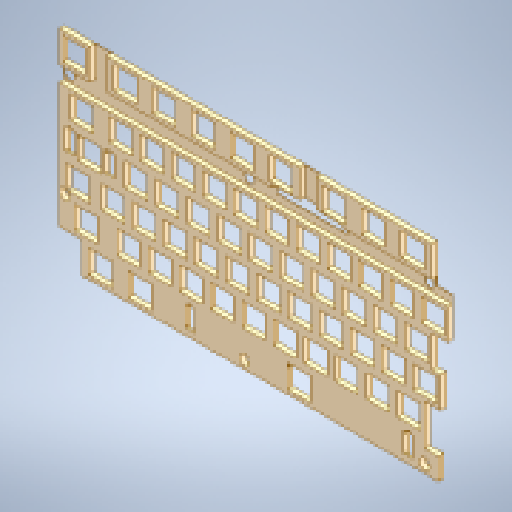
# Autodesk Inventor part: Left Plate
Saved by Autodesk Inventor 2025 (Build 290162000, 162)
## iProperties
Created: 2024-07-10
Part Number: Left Plate
Material: PET Plastic
Document SubType Name: Modeling
Designer: adam
Density: 1.541 g/cm^3
Appearance: Smooth - Off-White
Author: adam
Autodesk Inventor part; units mm, degrees
(part 1 of 3)
ref_plane "YZ Plane" through (0, 0, 0) normal (1, 0, 0) x (0, 1, 0)
ref_plane "XZ Plane" through (0, 0, 0) normal (0, 1, 0) x (-1, 0, 0)
ref_plane "XY Plane" through (0, 0, 0) normal (0, 0, 1) x (1, 0, 0)
sketch "Sketch5" plane through (0, 0, 0) normal (0, 0, 1) x (1, 0, 0)
  line L0 (-225, -62.5) -> (225, -62.5) construction
  line L1 (225, -62.5) -> (225, 62.5) construction
  line L2 (225, 62.5) -> (-225, 62.5) construction
  line L3 (-225, 62.5) -> (-225, -62.5) construction
  spline S0 degree 3 poles (89.83, -35.8909) (88.6584, -35.8909) (87.7087, -34.9412) (87.7087, -33.7696) knots 0 0 0 0 1 1 1 1 construction
  spline S1 degree 3 poles (87.7087, -33.7696) (87.7087, -32.598) (88.6584, -31.6483) (89.83, -31.6483) knots 0 0 0 0 1 1 1 1 construction
  arc A0 (91.9513, -33.7696) -> (89.83, -31.6483) centre (89.83, -33.7696) ccw construction
  spline S2 degree 3 poles (91.9513, -33.7696) (91.9513, -34.9412) (91.0016, -35.8909) (89.83, -35.8909) knots 0 0 0 0 1 1 1 1 construction
  arc A1 (215.8301, -43.274) -> (213.7088, -41.1527) centre (213.7088, -43.274) ccw construction
  spline S3 degree 3 poles (215.8301, -43.274) (215.8301, -44.4456) (214.8804, -45.3953) (213.7088, -45.3953) knots 0 0 0 0 1 1 1 1 construction
  spline S4 degree 3 poles (213.7088, -45.3953) (212.5372, -45.3953) (211.5875, -44.4456) (211.5875, -43.274) knots 0 0 0 0 1 1 1 1 construction
  spline S5 degree 3 poles (211.5875, -43.274) (211.5875, -42.1024) (212.5372, -41.1527) (213.7088, -41.1527) knots 0 0 0 0 1 1 1 1 construction
  arc A2 (196.7801, -33.722) -> (194.6588, -31.6007) centre (194.6588, -33.722) ccw construction
  spline S6 degree 3 poles (196.7801, -33.722) (196.7801, -34.58) (196.2633, -35.3535) (195.4706, -35.6818) knots 0 0 0 0 1 1 1 1 construction
  spline S7 degree 3 poles (195.4706, -35.6818) (194.6779, -36.0102) (193.7655, -35.8287) (193.1588, -35.222) knots 0 0 0 0 1 1 1 1 construction
  spline S8 degree 3 poles (193.1588, -35.222) (192.5521, -34.6153) (192.3706, -33.7029) (192.699, -32.9102) knots 0 0 0 0 1 1 1 1 construction
  spline S9 degree 3 poles (192.699, -32.9102) (193.0273, -32.1175) (193.8008, -31.6007) (194.6588, -31.6007) knots 0 0 0 0 1 1 1 1 construction
  arc A3 (196.7801, -52.772) -> (194.6588, -50.6507) centre (194.6588, -52.772) ccw construction
  spline S10 degree 3 poles (196.7801, -52.772) (196.7801, -53.63) (196.2633, -54.4035) (195.4706, -54.7318) knots 0 0 0 0 1 1 1 1 construction
  spline S11 degree 3 poles (195.4706, -54.7318) (194.6779, -55.0602) (193.7655, -54.8787) (193.1588, -54.272) knots 0 0 0 0 1 1 1 1 construction
  spline S12 degree 3 poles (193.1588, -54.272) (192.5521, -53.6653) (192.3706, -52.7529) (192.699, -51.9602) knots 0 0 0 0 1 1 1 1 construction
  spline S13 degree 3 poles (192.699, -51.9602) (193.0273, -51.1675) (193.8008, -50.6507) (194.6588, -50.6507) knots 0 0 0 0 1 1 1 1 construction
  arc A4 (215.8301, -14.672) -> (213.7088, -12.5507) centre (213.7088, -14.672) ccw construction
  spline S14 degree 3 poles (215.8301, -14.672) (215.8301, -15.53) (215.3133, -16.3035) (214.5206, -16.6318) knots 0 0 0 0 1 1 1 1 construction
  spline S15 degree 3 poles (214.5206, -16.6318) (213.7279, -16.9602) (212.8155, -16.7787) (212.2088, -16.172) knots 0 0 0 0 1 1 1 1 construction
  spline S16 degree 3 poles (212.2088, -16.172) (211.6021, -15.5653) (211.4206, -14.6529) (211.749, -13.8602) knots 0 0 0 0 1 1 1 1 construction
  spline S17 degree 3 poles (211.749, -13.8602) (212.0773, -13.0675) (212.8508, -12.5507) (213.7088, -12.5507) knots 0 0 0 0 1 1 1 1 construction
  arc A5 (196.7801, -14.672) -> (194.6588, -12.5507) centre (194.6588, -14.672) ccw construction
  spline S18 degree 3 poles (196.7801, -14.672) (196.7801, -15.53) (196.2633, -16.3035) (195.4706, -16.6318) knots 0 0 0 0 1 1 1 1 construction
  spline S19 degree 3 poles (195.4706, -16.6318) (194.6779, -16.9602) (193.7655, -16.7787) (193.1588, -16.172) knots 0 0 0 0 1 1 1 1 construction
  spline S20 degree 3 poles (193.1588, -16.172) (192.5521, -15.5653) (192.3706, -14.6529) (192.699, -13.8602) knots 0 0 0 0 1 1 1 1 construction
  spline S21 degree 3 poles (192.699, -13.8602) (193.0273, -13.0675) (193.8008, -12.5507) (194.6588, -12.5507) knots 0 0 0 0 1 1 1 1 construction
  spline S22 degree 3 poles (211.749, 5.1898) (212.0773, 5.9825) (212.8508, 6.4993) (213.7088, 6.4993) knots 0 0 0 0 1 1 1 1 construction
  arc A6 (215.8301, 4.378) -> (213.7088, 6.4993) centre (213.7088, 4.378) ccw construction
  spline S23 degree 3 poles (215.8301, 4.378) (215.8301, 3.52) (215.3133, 2.7465) (214.5206, 2.4182) knots 0 0 0 0 1 1 1 1 construction
  spline S24 degree 3 poles (214.5206, 2.4182) (213.7279, 2.0898) (212.8155, 2.2713) (212.2088, 2.878) knots 0 0 0 0 1 1 1 1 construction
  spline S25 degree 3 poles (212.2088, 2.878) (211.6021, 3.4847) (211.4206, 4.3971) (211.749, 5.1898) knots 0 0 0 0 1 1 1 1 construction
  arc A7 (196.7801, 4.378) -> (194.6588, 6.4993) centre (194.6588, 4.378) ccw construction
  spline S26 degree 3 poles (196.7801, 4.378) (196.7801, 3.52) (196.2633, 2.7465) (195.4706, 2.4182) knots 0 0 0 0 1 1 1 1 construction
  spline S27 degree 3 poles (195.4706, 2.4182) (194.6779, 2.0898) (193.7655, 2.2713) (193.1588, 2.878) knots 0 0 0 0 1 1 1 1 construction
  spline S28 degree 3 poles (193.1588, 2.878) (192.5521, 3.4847) (192.3706, 4.3971) (192.699, 5.1898) knots 0 0 0 0 1 1 1 1 construction
  spline S29 degree 3 poles (192.699, 5.1898) (193.0273, 5.9825) (193.8008, 6.4993) (194.6588, 6.4993) knots 0 0 0 0 1 1 1 1 construction
  spline S30 degree 3 poles (176.4206, 21.4682) (175.6279, 21.1398) (174.7155, 21.3213) (174.1088, 21.928) knots 0 0 0 0 1 1 1 1 construction
  spline S31 degree 3 poles (174.1088, 21.928) (173.5021, 22.5347) (173.3206, 23.4471) (173.649, 24.2398) knots 0 0 0 0 1 1 1 1 construction
  spline S32 degree 3 poles (173.649, 24.2398) (173.9773, 25.0325) (174.7508, 25.5493) (175.6088, 25.5493) knots 0 0 0 0 1 1 1 1 construction
  arc A8 (177.7301, 23.428) -> (175.6088, 25.5493) centre (175.6088, 23.428) ccw construction
  spline S33 degree 3 poles (177.7301, 23.428) (177.7301, 22.57) (177.2133, 21.7965) (176.4206, 21.4682) knots 0 0 0 0 1 1 1 1 construction
  spline S34 degree 3 poles (193.1588, 21.928) (192.5521, 22.5347) (192.3706, 23.4471) (192.699, 24.2398) knots 0 0 0 0 1 1 1 1 construction
  spline S35 degree 3 poles (192.699, 24.2398) (193.0273, 25.0325) (193.8008, 25.5493) (194.6588, 25.5493) knots 0 0 0 0 1 1 1 1 construction
  arc A9 (196.7801, 23.428) -> (194.6588, 25.5493) centre (194.6588, 23.428) ccw construction
  spline S36 degree 3 poles (196.7801, 23.428) (196.7801, 22.57) (196.2633, 21.7965) (195.4706, 21.4682) knots 0 0 0 0 1 1 1 1 construction
  spline S37 degree 3 poles (195.4706, 21.4682) (194.6779, 21.1398) (193.7655, 21.3213) (193.1588, 21.928) knots 0 0 0 0 1 1 1 1 construction
  arc A10 (215.8301, 23.428) -> (213.7088, 25.5493) centre (213.7088, 23.428) ccw construction
  spline S38 degree 3 poles (215.8301, 23.428) (215.8301, 22.57) (215.3133, 21.7965) (214.5206, 21.4682) knots 0 0 0 0 1 1 1 1 construction
  spline S39 degree 3 poles (214.5206, 21.4682) (213.7279, 21.1398) (212.8155, 21.3213) (212.2088, 21.928) knots 0 0 0 0 1 1 1 1 construction
  spline S40 degree 3 poles (212.2088, 21.928) (211.6021, 22.5347) (211.4206, 23.4471) (211.749, 24.2398) knots 0 0 0 0 1 1 1 1 construction
  spline S41 degree 3 poles (211.749, 24.2398) (212.0773, 25.0325) (212.8508, 25.5493) (213.7088, 25.5493) knots 0 0 0 0 1 1 1 1 construction
  arc A11 (168.3321, -52.772) -> (166.2108, -50.6507) centre (166.2108, -52.772) ccw construction
  spline S42 degree 3 poles (168.3321, -52.772) (168.3321, -53.63) (167.8153, -54.4035) (167.0226, -54.7318) knots 0 0 0 0 1 1 1 1 construction
  spline S43 degree 3 poles (167.0226, -54.7318) (166.2299, -55.0602) (165.3175, -54.8787) (164.7108, -54.272) knots 0 0 0 0 1 1 1 1 construction
  spline S44 degree 3 poles (164.7108, -54.272) (164.1041, -53.6653) (163.9226, -52.7529) (164.251, -51.9602) knots 0 0 0 0 1 1 1 1 construction
  spline S45 degree 3 poles (164.251, -51.9602) (164.5793, -51.1675) (165.3528, -50.6507) (166.2108, -50.6507) knots 0 0 0 0 1 1 1 1 construction
  arc A12 (177.7301, -33.722) -> (175.6088, -31.6007) centre (175.6088, -33.722) ccw construction
  spline S46 degree 3 poles (177.7301, -33.722) (177.7301, -34.58) (177.2133, -35.3535) (176.4206, -35.6818) knots 0 0 0 0 1 1 1 1 construction
  spline S47 degree 3 poles (176.4206, -35.6818) (175.6279, -36.0102) (174.7155, -35.8287) (174.1088, -35.222) knots 0 0 0 0 1 1 1 1 construction
  spline S48 degree 3 poles (174.1088, -35.222) (173.5021, -34.6153) (173.3206, -33.7029) (173.649, -32.9102) knots 0 0 0 0 1 1 1 1 construction
  spline S49 degree 3 poles (173.649, -32.9102) (173.9773, -32.1175) (174.7508, -31.6007) (175.6088, -31.6007) knots 0 0 0 0 1 1 1 1 construction
  arc A13 (158.6801, -33.722) -> (156.5588, -31.6007) centre (156.5588, -33.722) ccw construction
  spline S50 degree 3 poles (158.6801, -33.722) (158.6801, -34.58) (158.1633, -35.3535) (157.3706, -35.6818) knots 0 0 0 0 1 1 1 1 construction
  spline S51 degree 3 poles (157.3706, -35.6818) (156.5779, -36.0102) (155.6655, -35.8287) (155.0588, -35.222) knots 0 0 0 0 1 1 1 1 construction
  spline S52 degree 3 poles (155.0588, -35.222) (154.4521, -34.6153) (154.2706, -33.7029) (154.599, -32.9102) knots 0 0 0 0 1 1 1 1 construction
  spline S53 degree 3 poles (154.599, -32.9102) (154.9273, -32.1175) (155.7008, -31.6007) (156.5588, -31.6007) knots 0 0 0 0 1 1 1 1 construction
  spline S54 degree 3 poles (155.0588, 2.878) (154.4521, 3.4847) (154.2706, 4.3971) (154.599, 5.1898) knots 0 0 0 0 1 1 1 1 construction
  spline S55 degree 3 poles (154.599, 5.1898) (154.9273, 5.9825) (155.7008, 6.4993) (156.5588, 6.4993) knots 0 0 0 0 1 1 1 1 construction
  arc A14 (158.6801, 4.378) -> (156.5588, 6.4993) centre (156.5588, 4.378) ccw construction
  spline S56 degree 3 poles (158.6801, 4.378) (158.6801, 3.52) (158.1633, 2.7465) (157.3706, 2.4182) knots 0 0 0 0 1 1 1 1 construction
  spline S57 degree 3 poles (157.3706, 2.4182) (156.5779, 2.0898) (155.6655, 2.2713) (155.0588, 2.878) knots 0 0 0 0 1 1 1 1 construction
  spline S58 degree 3 poles (174.1088, 2.878) (173.5021, 3.4847) (173.3206, 4.3971) (173.649, 5.1898) knots 0 0 0 0 1 1 1 1 construction
  spline S59 degree 3 poles (173.649, 5.1898) (173.9773, 5.9825) (174.7508, 6.4993) (175.6088, 6.4993) knots 0 0 0 0 1 1 1 1 construction
  arc A15 (177.7301, 4.378) -> (175.6088, 6.4993) centre (175.6088, 4.378) ccw construction
  spline S60 degree 3 poles (177.7301, 4.378) (177.7301, 3.52) (177.2133, 2.7465) (176.4206, 2.4182) knots 0 0 0 0 1 1 1 1 construction
  spline S61 degree 3 poles (176.4206, 2.4182) (175.6279, 2.0898) (174.7155, 2.2713) (174.1088, 2.878) knots 0 0 0 0 1 1 1 1 construction
  spline S62 degree 3 poles (155.0588, -16.172) (154.4521, -15.5653) (154.2706, -14.6529) (154.599, -13.8602) knots 0 0 0 0 1 1 1 1 construction
  spline S63 degree 3 poles (154.599, -13.8602) (154.9273, -13.0675) (155.7008, -12.5507) (156.5588, -12.5507) knots 0 0 0 0 1 1 1 1 construction
  arc A16 (158.6801, -14.672) -> (156.5588, -12.5507) centre (156.5588, -14.672) ccw construction
  spline S64 degree 3 poles (158.6801, -14.672) (158.6801, -15.53) (158.1633, -16.3035) (157.3706, -16.6318) knots 0 0 0 0 1 1 1 1 construction
  spline S65 degree 3 poles (157.3706, -16.6318) (156.5779, -16.9602) (155.6655, -16.7787) (155.0588, -16.172) knots 0 0 0 0 1 1 1 1 construction
  arc A17 (177.7301, -14.672) -> (175.6088, -12.5507) centre (175.6088, -14.672) ccw construction
  spline S66 degree 3 poles (177.7301, -14.672) (177.7301, -15.53) (177.2133, -16.3035) (176.4206, -16.6318) knots 0 0 0 0 1 1 1 1 construction
  spline S67 degree 3 poles (176.4206, -16.6318) (175.6279, -16.9602) (174.7155, -16.7787) (174.1088, -16.172) knots 0 0 0 0 1 1 1 1 construction
  spline S68 degree 3 poles (174.1088, -16.172) (173.5021, -15.5653) (173.3206, -14.6529) (173.649, -13.8602) knots 0 0 0 0 1 1 1 1 construction
  spline S69 degree 3 poles (173.649, -13.8602) (173.9773, -13.0675) (174.7508, -12.5507) (175.6088, -12.5507) knots 0 0 0 0 1 1 1 1 construction
  arc A18 (158.6801, 23.428) -> (156.5588, 25.5493) centre (156.5588, 23.428) ccw construction
  spline S70 degree 3 poles (158.6801, 23.428) (158.6801, 22.57) (158.1633, 21.7965) (157.3706, 21.4682) knots 0 0 0 0 1 1 1 1 construction
  spline S71 degree 3 poles (157.3706, 21.4682) (156.5779, 21.1398) (155.6655, 21.3213) (155.0588, 21.928) knots 0 0 0 0 1 1 1 1 construction
  spline S72 degree 3 poles (155.0588, 21.928) (154.4521, 22.5347) (154.2706, 23.4471) (154.599, 24.2398) knots 0 0 0 0 1 1 1 1 construction
  spline S73 degree 3 poles (154.599, 24.2398) (154.9273, 25.0325) (155.7008, 25.5493) (156.5588, 25.5493) knots 0 0 0 0 1 1 1 1 construction
  spline S74 degree 3 poles (125.8087, -33.7696) (125.8087, -32.598) (126.7584, -31.6483) (127.93, -31.6483) knots 0 0 0 0 1 1 1 1 construction
  arc A19 (130.0513, -33.7696) -> (127.93, -31.6483) centre (127.93, -33.7696) ccw construction
  spline S75 degree 3 poles (130.0513, -33.7696) (130.0513, -34.9412) (129.1016, -35.8909) (127.93, -35.8909) knots 0 0 0 0 1 1 1 1 construction
  spline S76 degree 3 poles (127.93, -35.8909) (126.7584, -35.8909) (125.8087, -34.9412) (125.8087, -33.7696) knots 0 0 0 0 1 1 1 1 construction
  arc A20 (111.75, -57.5) -> (110, -55.75) centre (110, -57.5) ccw construction
  spline S77 degree 3 poles (111.75, -57.5) (111.75, -58.2078) (111.3236, -58.8459) (110.6697, -59.1168) knots 0 0 0 0 1 1 1 1 construction
  spline S78 degree 3 poles (110.6697, -59.1168) (110.0158, -59.3877) (109.2631, -59.2379) (108.7626, -58.7374) knots 0 0 0 0 1 1 1 1 construction
  spline S79 degree 3 poles (108.7626, -58.7374) (108.2621, -58.2369) (108.1123, -57.4842) (108.3832, -56.8303) knots 0 0 0 0 1 1 1 1 construction
  spline S80 degree 3 poles (108.3832, -56.8303) (108.6541, -56.1764) (109.2922, -55.75) (110, -55.75) knots 0 0 0 0 1 1 1 1 construction
  spline S81 degree 3 poles (121.654, 21.8944) (121.0473, 22.5011) (120.8658, 23.4135) (121.1942, 24.2062) knots 0 0 0 0 1 1 1 1 construction
  spline S82 degree 3 poles (121.1942, 24.2062) (121.5225, 24.9989) (122.296, 25.5157) (123.154, 25.5157) knots 0 0 0 0 1 1 1 1 construction
  arc A21 (125.2753, 23.3944) -> (123.154, 25.5157) centre (123.154, 23.3944) ccw construction
  spline S83 degree 3 poles (125.2753, 23.3944) (125.2753, 22.5364) (124.7585, 21.7629) (123.9658, 21.4346) knots 0 0 0 0 1 1 1 1 construction
  spline S84 degree 3 poles (123.9658, 21.4346) (123.1731, 21.1062) (122.2607, 21.2877) (121.654, 21.8944) knots 0 0 0 0 1 1 1 1 construction
  arc A22 (96.6793, 23.3944) -> (94.558, 25.5157) centre (94.558, 23.3944) ccw construction
  spline S85 degree 3 poles (96.6793, 23.3944) (96.6793, 22.5364) (96.1625, 21.7629) (95.3698, 21.4346) knots 0 0 0 0 1 1 1 1 construction
  spline S86 degree 3 poles (95.3698, 21.4346) (94.5771, 21.1062) (93.6647, 21.2877) (93.058, 21.8944) knots 0 0 0 0 1 1 1 1 construction
  spline S87 degree 3 poles (93.058, 21.8944) (92.4513, 22.5011) (92.2698, 23.4135) (92.5982, 24.2062) knots 0 0 0 0 1 1 1 1 construction
  spline S88 degree 3 poles (92.5982, 24.2062) (92.9265, 24.9989) (93.7, 25.5157) (94.558, 25.5157) knots 0 0 0 0 1 1 1 1 construction
  spline S89 degree 3 poles (107.38, -16.2196) (106.7733, -15.6129) (106.5918, -14.7005) (106.9202, -13.9078) knots 0 0 0 0 1 1 1 1 construction
  spline S90 degree 3 poles (106.9202, -13.9078) (107.2485, -13.1151) (108.022, -12.5983) (108.88, -12.5983) knots 0 0 0 0 1 1 1 1 construction
  arc A23 (111.0013, -14.7196) -> (108.88, -12.5983) centre (108.88, -14.7196) ccw construction
  spline S91 degree 3 poles (111.0013, -14.7196) (111.0013, -15.5776) (110.4845, -16.3511) (109.6918, -16.6794) knots 0 0 0 0 1 1 1 1 construction
  spline S92 degree 3 poles (109.6918, -16.6794) (108.8991, -17.0078) (107.9867, -16.8263) (107.38, -16.2196) knots 0 0 0 0 1 1 1 1 construction
  arc A24 (111.0013, -33.7696) -> (108.88, -31.6483) centre (108.88, -33.7696) ccw construction
  spline S93 degree 3 poles (111.0013, -33.7696) (111.0013, -34.6276) (110.4845, -35.4011) (109.6918, -35.7294) knots 0 0 0 0 1 1 1 1 construction
  spline S94 degree 3 poles (109.6918, -35.7294) (108.8991, -36.0578) (107.9867, -35.8763) (107.38, -35.2696) knots 0 0 0 0 1 1 1 1 construction
  spline S95 degree 3 poles (107.38, -35.2696) (106.7733, -34.6629) (106.5918, -33.7505) (106.9202, -32.9578) knots 0 0 0 0 1 1 1 1 construction
  spline S96 degree 3 poles (106.9202, -32.9578) (107.2485, -32.1651) (108.022, -31.6483) (108.88, -31.6483) knots 0 0 0 0 1 1 1 1 construction
  spline S97 degree 3 poles (40.947, 24.1414) (41.2753, 24.9341) (42.0488, 25.4509) (42.9068, 25.4509) knots 0 0 0 0 1 1 1 1 construction
  arc A25 (45.0281, 23.3296) -> (42.9068, 25.4509) centre (42.9068, 23.3296) ccw construction
  spline S98 degree 3 poles (45.0281, 23.3296) (45.0281, 22.4716) (44.5113, 21.6981) (43.7186, 21.3698) knots 0 0 0 0 1 1 1 1 construction
  spline S99 degree 3 poles (43.7186, 21.3698) (42.9259, 21.0414) (42.0135, 21.2229) (41.4068, 21.8296) knots 0 0 0 0 1 1 1 1 construction
  spline S100 degree 3 poles (41.4068, 21.8296) (40.8001, 22.4363) (40.6186, 23.3487) (40.947, 24.1414) knots 0 0 0 0 1 1 1 1 construction
  arc A26 (25.9781, 23.3296) -> (23.8568, 25.4509) centre (23.8568, 23.3296) ccw construction
  spline S101 degree 3 poles (25.9781, 23.3296) (25.9781, 22.4716) (25.4613, 21.6981) (24.6686, 21.3698) knots 0 0 0 0 1 1 1 1 construction
  spline S102 degree 3 poles (24.6686, 21.3698) (23.8759, 21.0414) (22.9635, 21.2229) (22.3568, 21.8296) knots 0 0 0 0 1 1 1 1 construction
  spline S103 degree 3 poles (22.3568, 21.8296) (21.7501, 22.4363) (21.5686, 23.3487) (21.897, 24.1414) knots 0 0 0 0 1 1 1 1 construction
  spline S104 degree 3 poles (21.897, 24.1414) (22.2253, 24.9341) (22.9988, 25.4509) (23.8568, 25.4509) knots 0 0 0 0 1 1 1 1 construction
  arc A27 (42.4881, 51.9864) -> (40.3668, 54.1077) centre (40.3668, 51.9864) ccw construction
  spline S105 degree 3 poles (42.4881, 51.9864) (42.4881, 50.8148) (41.5384, 49.8651) (40.3668, 49.8651) knots 0 0 0 0 1 1 1 1 construction
  spline S106 degree 3 poles (40.3668, 49.8651) (39.1952, 49.8651) (38.2455, 50.8148) (38.2455, 51.9864) knots 0 0 0 0 1 1 1 1 construction
  spline S107 degree 3 poles (38.2455, 51.9864) (38.2455, 53.158) (39.1952, 54.1077) (40.3668, 54.1077) knots 0 0 0 0 1 1 1 1 construction
  arc A28 (64.0781, 23.3296) -> (61.9568, 25.4509) centre (61.9568, 23.3296) ccw construction
  spline S108 degree 3 poles (64.0781, 23.3296) (64.0781, 22.158) (63.1284, 21.2083) (61.9568, 21.2083) knots 0 0 0 0 1 1 1 1 construction
  spline S109 degree 3 poles (61.9568, 21.2083) (60.7852, 21.2083) (59.8355, 22.158) (59.8355, 23.3296) knots 0 0 0 0 1 1 1 1 construction
  spline S110 degree 3 poles (59.8355, 23.3296) (59.8355, 24.5012) (60.7852, 25.4509) (61.9568, 25.4509) knots 0 0 0 0 1 1 1 1 construction
  spline S111 degree 3 poles (71.9023, 58.0219) (72.84, 57.0843) (73.3668, 55.8125) (73.3668, 54.4864) knots 0 0 0 0 1 1 1 1 construction
  spline S112 degree 3 poles (73.3668, 54.4864) (73.3668, 52.4641) (72.1486, 50.6409) (70.2802, 49.867) knots 0 0 0 0 1 1 1 1 construction
  spline S113 degree 3 poles (70.2802, 49.867) (68.4118, 49.0931) (66.2613, 49.5209) (64.8313, 50.9509) knots 0 0 0 0 1 1 1 1 construction
  spline S114 degree 3 poles (64.8313, 50.9509) (63.4013, 52.3809) (62.9735, 54.5314) (63.7474, 56.3998) knots 0 0 0 0 1 1 1 1 construction
  spline S115 degree 3 poles (63.7474, 56.3998) (64.5213, 58.2682) (66.3445, 59.4864) (68.3668, 59.4864) knots 0 0 0 0 1 1 1 1 construction
  spline S116 degree 3 poles (68.3668, 59.4864) (69.6929, 59.4864) (70.9647, 58.9596) (71.9023, 58.0219) knots 0 0 0 0 1 1 1 1 construction
  line L4 (54.4468, -24.8204) -> (60.4468, -24.8204) construction
  line L5 (60.4468, -24.8204) -> (60.4468, -39.8204) construction
  line L6 (60.4468, -39.8204) -> (54.4468, -39.8204) construction
  line L7 (54.4468, -39.8204) -> (54.4468, -24.8204) construction
  line L8 (50.6708, -14.3724) -> (65.6708, -14.3724) construction
  line L9 (65.6708, -14.3724) -> (65.6708, -20.3724) construction
  line L10 (65.6708, -20.3724) -> (50.6708, -20.3724) construction
  line L11 (50.6708, -20.3724) -> (50.6708, -14.3724) construction
  spline S117 degree 3 poles (-35.9979, -14.7704) (-35.9979, -15.6284) (-36.5147, -16.4019) (-37.3074, -16.7302) knots 0 0 0 0 1 1 1 1 construction
  spline S118 degree 3 poles (-37.3074, -16.7302) (-38.1001, -17.0586) (-39.0125, -16.8771) (-39.6192, -16.2704) knots 0 0 0 0 1 1 1 1 construction
  spline S119 degree 3 poles (-39.6192, -16.2704) (-40.2259, -15.6637) (-40.4074, -14.7513) (-40.079, -13.9586) knots 0 0 0 0 1 1 1 1 construction
  spline S120 degree 3 poles (-40.079, -13.9586) (-39.7507, -13.1659) (-38.9772, -12.6491) (-38.1192, -12.6491) knots 0 0 0 0 1 1 1 1 construction
  arc A29 (-35.9979, -14.7704) -> (-38.1192, -12.6491) centre (-38.1192, -14.7704) ccw construction
  spline S121 degree 3 poles (-26.3419, -33.8224) (-26.3419, -34.6804) (-26.8587, -35.4539) (-27.6514, -35.7822) knots 0 0 0 0 1 1 1 1 construction
  spline S122 degree 3 poles (-27.6514, -35.7822) (-28.4441, -36.1106) (-29.3565, -35.9291) (-29.9632, -35.3224) knots 0 0 0 0 1 1 1 1 construction
  spline S123 degree 3 poles (-29.9632, -35.3224) (-30.5699, -34.7157) (-30.7514, -33.8033) (-30.423, -33.0106) knots 0 0 0 0 1 1 1 1 construction
  spline S124 degree 3 poles (-30.423, -33.0106) (-30.0947, -32.2179) (-29.3212, -31.7011) (-28.4632, -31.7011) knots 0 0 0 0 1 1 1 1 construction
  spline S125 degree 3 poles (-28.4632, -31.7011) (-27.2916, -31.7011) (-26.3419, -32.6508) (-26.3419, -33.8224) knots 0 0 0 0 1 1 1 1 construction
  spline S126 degree 3 poles (-30.4494, 50.0266) (-31.2421, 49.6982) (-32.1545, 49.8797) (-32.7612, 50.4864) knots 0 0 0 0 1 1 1 1 construction
  spline S127 degree 3 poles (-32.7612, 50.4864) (-33.3679, 51.0931) (-33.5494, 52.0055) (-33.221, 52.7982) knots 0 0 0 0 1 1 1 1 construction
  spline S128 degree 3 poles (-33.221, 52.7982) (-32.8927, 53.5909) (-32.1192, 54.1077) (-31.2612, 54.1077) knots 0 0 0 0 1 1 1 1 construction
  arc A30 (-29.1399, 51.9864) -> (-31.2612, 54.1077) centre (-31.2612, 51.9864) ccw construction
  spline S129 degree 3 poles (-29.1399, 51.9864) (-29.1399, 51.1284) (-29.6567, 50.3549) (-30.4494, 50.0266) knots 0 0 0 0 1 1 1 1 construction
  spline S130 degree 3 poles (-31.1719, 23.3296) (-31.1719, 22.4716) (-31.6887, 21.6981) (-32.4814, 21.3698) knots 0 0 0 0 1 1 1 1 construction
  spline S131 degree 3 poles (-32.4814, 21.3698) (-33.2741, 21.0414) (-34.1865, 21.2229) (-34.7932, 21.8296) knots 0 0 0 0 1 1 1 1 construction
  spline S132 degree 3 poles (-34.7932, 21.8296) (-35.3999, 22.4363) (-35.5814, 23.3487) (-35.253, 24.1414) knots 0 0 0 0 1 1 1 1 construction
  spline S133 degree 3 poles (-35.253, 24.1414) (-34.9247, 24.9341) (-34.1512, 25.4509) (-33.2932, 25.4509) knots 0 0 0 0 1 1 1 1 construction
  arc A31 (-31.1719, 23.3296) -> (-33.2932, 25.4509) centre (-33.2932, 23.3296) ccw construction
  spline S134 degree 3 poles (-12.1219, 23.3296) (-12.1219, 22.4716) (-12.6387, 21.6981) (-13.4314, 21.3698) knots 0 0 0 0 1 1 1 1 construction
  spline S135 degree 3 poles (-13.4314, 21.3698) (-14.2241, 21.0414) (-15.1365, 21.2229) (-15.7432, 21.8296) knots 0 0 0 0 1 1 1 1 construction
  spline S136 degree 3 poles (-15.7432, 21.8296) (-16.3499, 22.4363) (-16.5314, 23.3487) (-16.203, 24.1414) knots 0 0 0 0 1 1 1 1 construction
  spline S137 degree 3 poles (-16.203, 24.1414) (-15.8747, 24.9341) (-15.1012, 25.4509) (-14.2432, 25.4509) knots 0 0 0 0 1 1 1 1 construction
  arc A32 (-12.1219, 23.3296) -> (-14.2432, 25.4509) centre (-14.2432, 23.3296) ccw construction
  arc A33 (-5.2639, 51.9864) -> (-7.3852, 54.1077) centre (-7.3852, 51.9864) ccw construction
  spline S138 degree 3 poles (-5.2639, 51.9864) (-5.2639, 51.1284) (-5.7807, 50.3549) (-6.5734, 50.0266) knots 0 0 0 0 1 1 1 1 construction
  spline S139 degree 3 poles (-6.5734, 50.0266) (-7.3661, 49.6982) (-8.2785, 49.8797) (-8.8852, 50.4864) knots 0 0 0 0 1 1 1 1 construction
  spline S140 degree 3 poles (-8.8852, 50.4864) (-9.4919, 51.0931) (-9.6734, 52.0055) (-9.345, 52.7982) knots 0 0 0 0 1 1 1 1 construction
  spline S141 degree 3 poles (-9.345, 52.7982) (-9.0167, 53.5909) (-8.2432, 54.1077) (-7.3852, 54.1077) knots 0 0 0 0 1 1 1 1 construction
  arc A34 (-2.7239, 4.2796) -> (-4.8452, 6.4009) centre (-4.8452, 4.2796) ccw construction
  spline S142 degree 3 poles (-2.7239, 4.2796) (-2.7239, 3.4216) (-3.2407, 2.6481) (-4.0334, 2.3198) knots 0 0 0 0 1 1 1 1 construction
  spline S143 degree 3 poles (-4.0334, 2.3198) (-4.8261, 1.9914) (-5.7385, 2.1729) (-6.3452, 2.7796) knots 0 0 0 0 1 1 1 1 construction
  spline S144 degree 3 poles (-6.3452, 2.7796) (-6.9519, 3.3863) (-7.1334, 4.2987) (-6.805, 5.0914) knots 0 0 0 0 1 1 1 1 construction
  spline S145 degree 3 poles (-6.805, 5.0914) (-6.4767, 5.8841) (-5.7032, 6.4009) (-4.8452, 6.4009) knots 0 0 0 0 1 1 1 1 construction
  arc A35 (-21.7739, 4.2796) -> (-23.8952, 6.4009) centre (-23.8952, 4.2796) ccw construction
  spline S146 degree 3 poles (-21.7739, 4.2796) (-21.7739, 3.4216) (-22.2907, 2.6481) (-23.0834, 2.3198) knots 0 0 0 0 1 1 1 1 construction
  spline S147 degree 3 poles (-23.0834, 2.3198) (-23.8761, 1.9914) (-24.7885, 2.1729) (-25.3952, 2.7796) knots 0 0 0 0 1 1 1 1 construction
  spline S148 degree 3 poles (-25.3952, 2.7796) (-26.0019, 3.3863) (-26.1834, 4.2987) (-25.855, 5.0914) knots 0 0 0 0 1 1 1 1 construction
  spline S149 degree 3 poles (-25.855, 5.0914) (-25.5267, 5.8841) (-24.7532, 6.4009) (-23.8952, 6.4009) knots 0 0 0 0 1 1 1 1 construction
  spline S150 degree 3 poles (-16.9479, -14.7704) (-16.9479, -15.6284) (-17.4647, -16.4019) (-18.2574, -16.7302) knots 0 0 0 0 1 1 1 1 construction
  spline S151 degree 3 poles (-18.2574, -16.7302) (-19.0501, -17.0586) (-19.9625, -16.8771) (-20.5692, -16.2704) knots 0 0 0 0 1 1 1 1 construction
  spline S152 degree 3 poles (-20.5692, -16.2704) (-21.1759, -15.6637) (-21.3574, -14.7513) (-21.029, -13.9586) knots 0 0 0 0 1 1 1 1 construction
  spline S153 degree 3 poles (-21.029, -13.9586) (-20.7007, -13.1659) (-19.9272, -12.6491) (-19.0692, -12.6491) knots 0 0 0 0 1 1 1 1 construction
  arc A36 (-16.9479, -14.7704) -> (-19.0692, -12.6491) centre (-19.0692, -14.7704) ccw construction
  spline S154 degree 3 poles (2.3561, -14.7704) (2.3561, -15.6284) (1.8393, -16.4019) (1.0466, -16.7302) knots 0 0 0 0 1 1 1 1 construction
  spline S155 degree 3 poles (1.0466, -16.7302) (0.2539, -17.0586) (-0.6585, -16.8771) (-1.2652, -16.2704) knots 0 0 0 0 1 1 1 1 construction
  spline S156 degree 3 poles (-1.2652, -16.2704) (-1.8719, -15.6637) (-2.0534, -14.7513) (-1.725, -13.9586) knots 0 0 0 0 1 1 1 1 construction
  spline S157 degree 3 poles (-1.725, -13.9586) (-1.3967, -13.1659) (-0.6232, -12.6491) (0.2348, -12.6491) knots 0 0 0 0 1 1 1 1 construction
  arc A37 (2.3561, -14.7704) -> (0.2348, -12.6491) centre (0.2348, -14.7704) ccw construction
  arc A38 (-7.3019, -33.8424) -> (-9.4232, -31.7211) centre (-9.4232, -33.8424) ccw construction
  spline S158 degree 3 poles (-7.3019, -33.8424) (-7.3019, -34.7004) (-7.8187, -35.4739) (-8.6114, -35.8022) knots 0 0 0 0 1 1 1 1 construction
  spline S159 degree 3 poles (-8.6114, -35.8022) (-9.4041, -36.1306) (-10.3165, -35.9491) (-10.9232, -35.3424) knots 0 0 0 0 1 1 1 1 construction
  spline S160 degree 3 poles (-10.9232, -35.3424) (-11.5299, -34.7357) (-11.7114, -33.8233) (-11.383, -33.0306) knots 0 0 0 0 1 1 1 1 construction
  spline S161 degree 3 poles (-11.383, -33.0306) (-11.0547, -32.2379) (-10.2812, -31.7211) (-9.4232, -31.7211) knots 0 0 0 0 1 1 1 1 construction
  line L12 (-6.8755, -43.9454) -> (-6.8755, -58.9454) construction
  line L13 (-6.8755, -58.9454) -> (-12.8755, -58.9454) construction
  line L14 (-12.8755, -58.9454) -> (-12.8755, -43.9454) construction
  line L15 (-12.8755, -43.9454) -> (-6.8755, -43.9454) construction
  spline S162 degree 3 poles (-1.6168, 38.3081) (-1.3459, 38.962) (-0.7078, 39.3884) (0, 39.3884) knots 0 0 0 0 1 1 1 1 construction
  arc A39 (1.75, 37.6384) -> (0, 39.3884) centre (0, 37.6384) ccw construction
  spline S163 degree 3 poles (1.75, 37.6384) (1.75, 36.9306) (1.3236, 36.2925) (0.6697, 36.0216) knots 0 0 0 0 1 1 1 1 construction
  spline S164 degree 3 poles (0.6697, 36.0216) (0.0158, 35.7507) (-0.7369, 35.9005) (-1.2374, 36.401) knots 0 0 0 0 1 1 1 1 construction
  spline S165 degree 3 poles (-1.2374, 36.401) (-1.7379, 36.9015) (-1.8877, 37.6542) (-1.6168, 38.3081) knots 0 0 0 0 1 1 1 1 construction
  spline S166 degree 3 poles (1.75, -57.5) (1.75, -58.2078) (1.3236, -58.8459) (0.6697, -59.1168) knots 0 0 0 0 1 1 1 1 construction
  spline S167 degree 3 poles (0.6697, -59.1168) (0.0158, -59.3877) (-0.7369, -59.2379) (-1.2374, -58.7374) knots 0 0 0 0 1 1 1 1 construction
  spline S168 degree 3 poles (-1.2374, -58.7374) (-1.7379, -58.2369) (-1.8877, -57.4842) (-1.6168, -56.8303) knots 0 0 0 0 1 1 1 1 construction
  spline S169 degree 3 poles (-1.6168, -56.8303) (-1.3459, -56.1764) (-0.7078, -55.75) (0, -55.75) knots 0 0 0 0 1 1 1 1 construction
  arc A40 (1.75, -57.5) -> (0, -55.75) centre (0, -57.5) ccw construction
  arc A41 (6.9281, 23.3296) -> (4.8068, 25.4509) centre (4.8068, 23.3296) ccw construction
  spline S170 degree 3 poles (6.9281, 23.3296) (6.9281, 22.4716) (6.4113, 21.6981) (5.6186, 21.3698) knots 0 0 0 0 1 1 1 1 construction
  spline S171 degree 3 poles (5.6186, 21.3698) (4.8259, 21.0414) (3.9135, 21.2229) (3.3068, 21.8296) knots 0 0 0 0 1 1 1 1 construction
  spline S172 degree 3 poles (3.3068, 21.8296) (2.7001, 22.4363) (2.5186, 23.3487) (2.847, 24.1414) knots 0 0 0 0 1 1 1 1 construction
  spline S173 degree 3 poles (2.847, 24.1414) (3.1753, 24.9341) (3.9488, 25.4509) (4.8068, 25.4509) knots 0 0 0 0 1 1 1 1 construction
  spline S174 degree 3 poles (14.531, 52.7982) (14.8593, 53.5909) (15.6328, 54.1077) (16.4908, 54.1077) knots 0 0 0 0 1 1 1 1 construction
  arc A42 (18.6121, 51.9864) -> (16.4908, 54.1077) centre (16.4908, 51.9864) ccw construction
  spline S175 degree 3 poles (18.6121, 51.9864) (18.6121, 51.1284) (18.0953, 50.3549) (17.3026, 50.0266) knots 0 0 0 0 1 1 1 1 construction
  spline S176 degree 3 poles (17.3026, 50.0266) (16.5099, 49.6982) (15.5975, 49.8797) (14.9908, 50.4864) knots 0 0 0 0 1 1 1 1 construction
  spline S177 degree 3 poles (14.9908, 50.4864) (14.3841, 51.0931) (14.2026, 52.0055) (14.531, 52.7982) knots 0 0 0 0 1 1 1 1 construction
  spline S178 degree 3 poles (8.1328, -35.3204) (7.5261, -34.7137) (7.3446, -33.8013) (7.673, -33.0086) knots 0 0 0 0 1 1 1 1 construction
  spline S179 degree 3 poles (7.673, -33.0086) (8.0013, -32.2159) (8.7748, -31.6991) (9.6328, -31.6991) knots 0 0 0 0 1 1 1 1 construction
  arc A43 (11.7541, -33.8204) -> (9.6328, -31.6991) centre (9.6328, -33.8204) ccw construction
  spline S180 degree 3 poles (11.7541, -33.8204) (11.7541, -34.6784) (11.2373, -35.4519) (10.4446, -35.7802) knots 0 0 0 0 1 1 1 1 construction
  spline S181 degree 3 poles (10.4446, -35.7802) (9.6519, -36.1086) (8.7395, -35.9271) (8.1328, -35.3204) knots 0 0 0 0 1 1 1 1 construction
  spline S182 degree 3 poles (36.2135, -14.7704) (36.2135, -13.5988) (37.1632, -12.6491) (38.3348, -12.6491) knots 0 0 0 0 1 1 1 1 construction
  arc A44 (40.4561, -14.7704) -> (38.3348, -12.6491) centre (38.3348, -14.7704) ccw construction
  spline S183 degree 3 poles (40.4561, -14.7704) (40.4561, -15.942) (39.5064, -16.8917) (38.3348, -16.8917) knots 0 0 0 0 1 1 1 1 construction
  spline S184 degree 3 poles (38.3348, -16.8917) (37.1632, -16.8917) (36.2135, -15.942) (36.2135, -14.7704) knots 0 0 0 0 1 1 1 1 construction
  spline S185 degree 3 poles (17.7848, -16.2704) (17.1781, -15.6637) (16.9966, -14.7513) (17.325, -13.9586) knots 0 0 0 0 1 1 1 1 construction
  spline S186 degree 3 poles (17.325, -13.9586) (17.6533, -13.1659) (18.4268, -12.6491) (19.2848, -12.6491) knots 0 0 0 0 1 1 1 1 construction
  arc A45 (21.4061, -14.7704) -> (19.2848, -12.6491) centre (19.2848, -14.7704) ccw construction
  spline S187 degree 3 poles (21.4061, -14.7704) (21.4061, -15.6284) (20.8893, -16.4019) (20.0966, -16.7302) knots 0 0 0 0 1 1 1 1 construction
  spline S188 degree 3 poles (20.0966, -16.7302) (19.3039, -17.0586) (18.3915, -16.8771) (17.7848, -16.2704) knots 0 0 0 0 1 1 1 1 construction
  arc A46 (16.3261, 4.2796) -> (14.2048, 6.4009) centre (14.2048, 4.2796) ccw construction
  spline S189 degree 3 poles (16.3261, 4.2796) (16.3261, 3.4216) (15.8093, 2.6481) (15.0166, 2.3198) knots 0 0 0 0 1 1 1 1 construction
  spline S190 degree 3 poles (15.0166, 2.3198) (14.2239, 1.9914) (13.3115, 2.1729) (12.7048, 2.7796) knots 0 0 0 0 1 1 1 1 construction
  spline S191 degree 3 poles (12.7048, 2.7796) (12.0981, 3.3863) (11.9166, 4.2987) (12.245, 5.0914) knots 0 0 0 0 1 1 1 1 construction
  spline S192 degree 3 poles (12.245, 5.0914) (12.5733, 5.8841) (13.3468, 6.4009) (14.2048, 6.4009) knots 0 0 0 0 1 1 1 1 construction
  arc A47 (35.3761, 4.2796) -> (33.2548, 6.4009) centre (33.2548, 4.2796) ccw construction
  spline S193 degree 3 poles (35.3761, 4.2796) (35.3761, 3.4216) (34.8593, 2.6481) (34.0666, 2.3198) knots 0 0 0 0 1 1 1 1 construction
  spline S194 degree 3 poles (34.0666, 2.3198) (33.2739, 1.9914) (32.3615, 2.1729) (31.7548, 2.7796) knots 0 0 0 0 1 1 1 1 construction
  spline S195 degree 3 poles (31.7548, 2.7796) (31.1481, 3.3863) (30.9666, 4.2987) (31.295, 5.0914) knots 0 0 0 0 1 1 1 1 construction
  spline S196 degree 3 poles (31.295, 5.0914) (31.6233, 5.8841) (32.3968, 6.4009) (33.2548, 6.4009) knots 0 0 0 0 1 1 1 1 construction
  arc A48 (61.7921, -5.3724) -> (59.6708, -3.2511) centre (59.6708, -5.3724) ccw construction
  spline S197 degree 3 poles (61.7921, -5.3724) (61.7921, -6.2304) (61.2753, -7.0039) (60.4826, -7.3322) knots 0 0 0 0 1 1 1 1 construction
  spline S198 degree 3 poles (60.4826, -7.3322) (59.6899, -7.6606) (58.7775, -7.4791) (58.1708, -6.8724) knots 0 0 0 0 1 1 1 1 construction
  spline S199 degree 3 poles (58.1708, -6.8724) (57.5641, -6.2657) (57.3826, -5.3533) (57.711, -4.5606) knots 0 0 0 0 1 1 1 1 construction
  spline S200 degree 3 poles (57.711, -4.5606) (58.0393, -3.7679) (58.8128, -3.2511) (59.6708, -3.2511) knots 0 0 0 0 1 1 1 1 construction
  spline S201 degree 3 poles (23.1841, -52.8704) (23.1841, -53.7284) (22.6673, -54.5019) (21.8746, -54.8302) knots 0 0 0 0 1 1 1 1 construction
  spline S202 degree 3 poles (21.8746, -54.8302) (21.0819, -55.1586) (20.1695, -54.9771) (19.5628, -54.3704) knots 0 0 0 0 1 1 1 1 construction
  spline S203 degree 3 poles (19.5628, -54.3704) (18.9561, -53.7637) (18.7746, -52.8513) (19.103, -52.0586) knots 0 0 0 0 1 1 1 1 construction
  spline S204 degree 3 poles (19.103, -52.0586) (19.4313, -51.2659) (20.2048, -50.7491) (21.0628, -50.7491) knots 0 0 0 0 1 1 1 1 construction
  arc A49 (23.1841, -52.8704) -> (21.0628, -50.7491) centre (21.0628, -52.8704) ccw construction
  line L16 (36.4468, -24.8204) -> (36.4468, -39.8204) construction
  line L17 (36.4468, -39.8204) -> (30.4468, -39.8204) construction
  line L18 (30.4468, -39.8204) -> (30.4468, -24.8204) construction
  line L19 (30.4468, -24.8204) -> (36.4468, -24.8204) construction
  spline S205 degree 3 poles (47.0601, -52.8704) (47.0601, -54.042) (46.1104, -54.9917) (44.9388, -54.9917) knots 0 0 0 0 1 1 1 1 construction
  spline S206 degree 3 poles (44.9388, -54.9917) (43.7672, -54.9917) (42.8175, -54.042) (42.8175, -52.8704) knots 0 0 0 0 1 1 1 1 construction
  spline S207 degree 3 poles (42.8175, -52.8704) (42.8175, -51.6988) (43.7672, -50.7491) (44.9388, -50.7491) knots 0 0 0 0 1 1 1 1 construction
  arc A50 (47.0601, -52.8704) -> (44.9388, -50.7491) centre (44.9388, -52.8704) ccw construction
  spline S208 degree 3 poles (-154.5405, -14.7704) (-154.5405, -13.5988) (-153.5908, -12.6491) (-152.4192, -12.6491) knots 0 0 0 0 1 1 1 1 construction
  arc A51 (-150.2979, -14.7704) -> (-152.4192, -12.6491) centre (-152.4192, -14.7704) ccw construction
  spline S209 degree 3 poles (-150.2979, -14.7704) (-150.2979, -15.942) (-151.2476, -16.8917) (-152.4192, -16.8917) knots 0 0 0 0 1 1 1 1 construction
  spline S210 degree 3 poles (-152.4192, -16.8917) (-153.5908, -16.8917) (-154.5405, -15.942) (-154.5405, -14.7704) knots 0 0 0 0 1 1 1 1 construction
  spline S211 degree 3 poles (-172.9692, -16.2704) (-173.5759, -15.6637) (-173.7574, -14.7513) (-173.429, -13.9586) knots 0 0 0 0 1 1 1 1 construction
  spline S212 degree 3 poles (-173.429, -13.9586) (-173.1007, -13.1659) (-172.3272, -12.6491) (-171.4692, -12.6491) knots 0 0 0 0 1 1 1 1 construction
  arc A52 (-169.3479, -14.7704) -> (-171.4692, -12.6491) centre (-171.4692, -14.7704) ccw construction
  spline S213 degree 3 poles (-169.3479, -14.7704) (-169.3479, -15.6284) (-169.8647, -16.4019) (-170.6574, -16.7302) knots 0 0 0 0 1 1 1 1 construction
  spline S214 degree 3 poles (-170.6574, -16.7302) (-171.4501, -17.0586) (-172.3625, -16.8771) (-172.9692, -16.2704) knots 0 0 0 0 1 1 1 1 construction
  spline S215 degree 3 poles (-163.9385, -33.8204) (-163.9385, -32.6488) (-162.9888, -31.6991) (-161.8172, -31.6991) knots 0 0 0 0 1 1 1 1 construction
  arc A53 (-159.6959, -33.8204) -> (-161.8172, -31.6991) centre (-161.8172, -33.8204) ccw construction
  spline S216 degree 3 poles (-159.6959, -33.8204) (-159.6959, -34.992) (-160.6456, -35.9417) (-161.8172, -35.9417) knots 0 0 0 0 1 1 1 1 construction
  spline S217 degree 3 poles (-161.8172, -35.9417) (-162.9888, -35.9417) (-163.9385, -34.992) (-163.9385, -33.8204) knots 0 0 0 0 1 1 1 1 construction
  arc A54 (-172.1419, -52.8704) -> (-174.2632, -50.7491) centre (-174.2632, -52.8704) ccw construction
  spline S218 degree 3 poles (-172.1419, -52.8704) (-172.1419, -53.7284) (-172.6587, -54.5019) (-173.4514, -54.8302) knots 0 0 0 0 1 1 1 1 construction
  spline S219 degree 3 poles (-173.4514, -54.8302) (-174.2441, -55.1586) (-175.1565, -54.9771) (-175.7632, -54.3704) knots 0 0 0 0 1 1 1 1 construction
  spline S220 degree 3 poles (-175.7632, -54.3704) (-176.3699, -53.7637) (-176.5514, -52.8513) (-176.223, -52.0586) knots 0 0 0 0 1 1 1 1 construction
  spline S221 degree 3 poles (-176.223, -52.0586) (-175.8947, -51.2659) (-175.1212, -50.7491) (-174.2632, -50.7491) knots 0 0 0 0 1 1 1 1 construction
  arc A55 (-178.7459, -33.8204) -> (-180.8672, -31.6991) centre (-180.8672, -33.8204) ccw construction
  spline S222 degree 3 poles (-178.7459, -33.8204) (-178.7459, -34.6784) (-179.2627, -35.4519) (-180.0554, -35.7802) knots 0 0 0 0 1 1 1 1 construction
  spline S223 degree 3 poles (-180.0554, -35.7802) (-180.8481, -36.1086) (-181.7605, -35.9271) (-182.3672, -35.3204) knots 0 0 0 0 1 1 1 1 construction
  spline S224 degree 3 poles (-182.3672, -35.3204) (-182.9739, -34.7137) (-183.1554, -33.8013) (-182.827, -33.0086) knots 0 0 0 0 1 1 1 1 construction
  spline S225 degree 3 poles (-182.827, -33.0086) (-182.4987, -32.2159) (-181.7252, -31.6991) (-180.8672, -31.6991) knots 0 0 0 0 1 1 1 1 construction
  spline S226 degree 3 poles (-204.9079, -33.8204) (-204.9079, -34.6784) (-205.4247, -35.4519) (-206.2174, -35.7802) knots 0 0 0 0 1 1 1 1 construction
  spline S227 degree 3 poles (-206.2174, -35.7802) (-207.0101, -36.1086) (-207.9225, -35.9271) (-208.5292, -35.3204) knots 0 0 0 0 1 1 1 1 construction
  spline S228 degree 3 poles (-208.5292, -35.3204) (-209.1359, -34.7137) (-209.3174, -33.8013) (-208.989, -33.0086) knots 0 0 0 0 1 1 1 1 construction
  spline S229 degree 3 poles (-208.989, -33.0086) (-208.6607, -32.2159) (-207.8872, -31.6991) (-207.0292, -31.6991) knots 0 0 0 0 1 1 1 1 construction
  arc A56 (-204.9079, -33.8204) -> (-207.0292, -31.6991) centre (-207.0292, -33.8204) ccw construction
  arc A57 (-218.25, -24.5) -> (-220, -22.75) centre (-220, -24.5) ccw construction
  spline S230 degree 3 poles (-218.25, -24.5) (-218.25, -25.2078) (-218.6764, -25.8459) (-219.3303, -26.1168) knots 0 0 0 0 1 1 1 1 construction
  spline S231 degree 3 poles (-219.3303, -26.1168) (-219.9842, -26.3877) (-220.7369, -26.2379) (-221.2374, -25.7374) knots 0 0 0 0 1 1 1 1 construction
  spline S232 degree 3 poles (-221.2374, -25.7374) (-221.7379, -25.2369) (-221.8877, -24.4842) (-221.6168, -23.8303) knots 0 0 0 0 1 1 1 1 construction
  spline S233 degree 3 poles (-221.6168, -23.8303) (-221.3459, -23.1764) (-220.7078, -22.75) (-220, -22.75) knots 0 0 0 0 1 1 1 1 construction
  arc A58 (-180.9715, 52.1016) -> (-183.0928, 54.2229) centre (-183.0928, 52.1016) ccw construction
  spline S234 degree 3 poles (-180.9715, 52.1016) (-180.9715, 51.2436) (-181.4883, 50.4701) (-182.281, 50.1418) knots 0 0 0 0 1 1 1 1 construction
  spline S235 degree 3 poles (-182.281, 50.1418) (-183.0737, 49.8134) (-183.9861, 49.9949) (-184.5928, 50.6016) knots 0 0 0 0 1 1 1 1 construction
  spline S236 degree 3 poles (-184.5928, 50.6016) (-185.1995, 51.2083) (-185.381, 52.1207) (-185.0526, 52.9134) knots 0 0 0 0 1 1 1 1 construction
  spline S237 degree 3 poles (-185.0526, 52.9134) (-184.7243, 53.7061) (-183.9508, 54.2229) (-183.0928, 54.2229) knots 0 0 0 0 1 1 1 1 construction
  arc A59 (-212.0199, 51.8884) -> (-214.1412, 54.0097) centre (-214.1412, 51.8884) ccw construction
  spline S238 degree 3 poles (-212.0199, 51.8884) (-212.0199, 51.0304) (-212.5367, 50.2569) (-213.3294, 49.9286) knots 0 0 0 0 1 1 1 1 construction
  spline S239 degree 3 poles (-213.3294, 49.9286) (-214.1221, 49.6002) (-215.0345, 49.7817) (-215.6412, 50.3884) knots 0 0 0 0 1 1 1 1 construction
  spline S240 degree 3 poles (-215.6412, 50.3884) (-216.2479, 50.9951) (-216.4294, 51.9075) (-216.101, 52.7002) knots 0 0 0 0 1 1 1 1 construction
  spline S241 degree 3 poles (-216.101, 52.7002) (-215.7727, 53.4929) (-214.9992, 54.0097) (-214.1412, 54.0097) knots 0 0 0 0 1 1 1 1 construction
  arc A60 (-218.25, 37.6384) -> (-220, 39.3884) centre (-220, 37.6384) ccw construction
  spline S242 degree 3 poles (-218.25, 37.6384) (-218.25, 36.9306) (-218.6764, 36.2925) (-219.3303, 36.0216) knots 0 0 0 0 1 1 1 1 construction
  spline S243 degree 3 poles (-219.3303, 36.0216) (-219.9842, 35.7507) (-220.7369, 35.9005) (-221.2374, 36.401) knots 0 0 0 0 1 1 1 1 construction
  spline S244 degree 3 poles (-221.2374, 36.401) (-221.7379, 36.9015) (-221.8877, 37.6542) (-221.6168, 38.3081) knots 0 0 0 0 1 1 1 1 construction
  spline S245 degree 3 poles (-221.6168, 38.3081) (-221.3459, 38.962) (-220.7078, 39.3884) (-220, 39.3884) knots 0 0 0 0 1 1 1 1 construction
  spline S246 degree 3 poles (-209.7339, -14.7704) (-209.7339, -15.6284) (-210.2507, -16.4019) (-211.0434, -16.7302) knots 0 0 0 0 1 1 1 1 construction
  spline S247 degree 3 poles (-211.0434, -16.7302) (-211.8361, -17.0586) (-212.7485, -16.8771) (-213.3552, -16.2704) knots 0 0 0 0 1 1 1 1 construction
  spline S248 degree 3 poles (-213.3552, -16.2704) (-213.9619, -15.6637) (-214.1434, -14.7513) (-213.815, -13.9586) knots 0 0 0 0 1 1 1 1 construction
  spline S249 degree 3 poles (-213.815, -13.9586) (-213.4867, -13.1659) (-212.7132, -12.6491) (-211.8552, -12.6491) knots 0 0 0 0 1 1 1 1 construction
  arc A61 (-209.7339, -14.7704) -> (-211.8552, -12.6491) centre (-211.8552, -14.7704) ccw construction
  spline S250 degree 3 poles (-190.5192, -12.6491) (-189.3476, -12.6491) (-188.3979, -13.5988) (-188.3979, -14.7704) knots 0 0 0 0 1 1 1 1 construction
  spline S251 degree 3 poles (-188.3979, -14.7704) (-188.3979, -15.6284) (-188.9147, -16.4019) (-189.7074, -16.7302) knots 0 0 0 0 1 1 1 1 construction
  spline S252 degree 3 poles (-189.7074, -16.7302) (-190.5001, -17.0586) (-191.4125, -16.8771) (-192.0192, -16.2704) knots 0 0 0 0 1 1 1 1 construction
  spline S253 degree 3 poles (-192.0192, -16.2704) (-192.6259, -15.6637) (-192.8074, -14.7513) (-192.479, -13.9586) knots 0 0 0 0 1 1 1 1 construction
  spline S254 degree 3 poles (-192.479, -13.9586) (-192.1507, -13.1659) (-191.3772, -12.6491) (-190.5192, -12.6491) knots 0 0 0 0 1 1 1 1 construction
  spline S255 degree 3 poles (-202.6219, 4.2796) (-202.6219, 3.4216) (-203.1387, 2.6481) (-203.9314, 2.3198) knots 0 0 0 0 1 1 1 1 construction
  spline S256 degree 3 poles (-203.9314, 2.3198) (-204.7241, 1.9914) (-205.6365, 2.1729) (-206.2432, 2.7796) knots 0 0 0 0 1 1 1 1 construction
  spline S257 degree 3 poles (-206.2432, 2.7796) (-206.8499, 3.3863) (-207.0314, 4.2987) (-206.703, 5.0914) knots 0 0 0 0 1 1 1 1 construction
  spline S258 degree 3 poles (-206.703, 5.0914) (-206.3747, 5.8841) (-205.6012, 6.4009) (-204.7432, 6.4009) knots 0 0 0 0 1 1 1 1 construction
  arc A62 (-202.6219, 4.2796) -> (-204.7432, 6.4009) centre (-204.7432, 4.2796) ccw construction
  spline S259 degree 3 poles (-207.3499, 23.3296) (-207.3499, 22.158) (-208.2996, 21.2083) (-209.4712, 21.2083) knots 0 0 0 0 1 1 1 1 construction
  spline S260 degree 3 poles (-209.4712, 21.2083) (-210.6428, 21.2083) (-211.5925, 22.158) (-211.5925, 23.3296) knots 0 0 0 0 1 1 1 1 construction
  spline S261 degree 3 poles (-211.5925, 23.3296) (-211.5925, 24.5012) (-210.6428, 25.4509) (-209.4712, 25.4509) knots 0 0 0 0 1 1 1 1 construction
  arc A63 (-207.3499, 23.3296) -> (-209.4712, 25.4509) centre (-209.4712, 23.3296) ccw construction
  line L20 (-219.7432, -1.7204) -> (-219.7432, 13.2796) construction
  line L21 (-219.7432, 13.2796) -> (-213.7432, 13.2796) construction
  line L22 (-213.7432, 13.2796) -> (-213.7432, -1.7204) construction
  line L23 (-213.7432, -1.7204) -> (-219.7432, -1.7204) construction
  line L24 (-195.7432, -1.7204) -> (-195.7432, 13.2796) construction
  line L25 (-195.7432, 13.2796) -> (-189.7432, 13.2796) construction
  line L26 (-189.7432, 13.2796) -> (-189.7432, -1.7204) construction
  line L27 (-189.7432, -1.7204) -> (-195.7432, -1.7204) construction
  spline S262 degree 3 poles (-197.3274, -54.8302) (-198.1201, -55.1586) (-199.0325, -54.9771) (-199.6392, -54.3704) knots 0 0 0 0 1 1 1 1 construction
  spline S263 degree 3 poles (-199.6392, -54.3704) (-200.2459, -53.7637) (-200.4274, -52.8513) (-200.099, -52.0586) knots 0 0 0 0 1 1 1 1 construction
  spline S264 degree 3 poles (-200.099, -52.0586) (-199.7707, -51.2659) (-198.9972, -50.7491) (-198.1392, -50.7491) knots 0 0 0 0 1 1 1 1 construction
  arc A64 (-196.0179, -52.8704) -> (-198.1392, -50.7491) centre (-198.1392, -52.8704) ccw construction
  spline S265 degree 3 poles (-196.0179, -52.8704) (-196.0179, -53.7284) (-196.5347, -54.5019) (-197.3274, -54.8302) knots 0 0 0 0 1 1 1 1 construction
  spline S266 degree 3 poles (-168.603, 24.1414) (-168.2747, 24.9341) (-167.5012, 25.4509) (-166.6432, 25.4509) knots 0 0 0 0 1 1 1 1 construction
  spline S267 degree 3 poles (-166.6432, 25.4509) (-165.4716, 25.4509) (-164.5219, 24.5012) (-164.5219, 23.3296) knots 0 0 0 0 1 1 1 1 construction
  spline S268 degree 3 poles (-164.5219, 23.3296) (-164.5219, 22.4716) (-165.0387, 21.6981) (-165.8314, 21.3698) knots 0 0 0 0 1 1 1 1 construction
  spline S269 degree 3 poles (-165.8314, 21.3698) (-166.6241, 21.0414) (-167.5365, 21.2229) (-168.1432, 21.8296) knots 0 0 0 0 1 1 1 1 construction
  spline S270 degree 3 poles (-168.1432, 21.8296) (-168.7499, 22.4363) (-168.9314, 23.3487) (-168.603, 24.1414) knots 0 0 0 0 1 1 1 1 construction
  spline S271 degree 3 poles (-187.1932, 21.8296) (-187.7999, 22.4363) (-187.9814, 23.3487) (-187.653, 24.1414) knots 0 0 0 0 1 1 1 1 construction
  spline S272 degree 3 poles (-187.653, 24.1414) (-187.3247, 24.9341) (-186.5512, 25.4509) (-185.6932, 25.4509) knots 0 0 0 0 1 1 1 1 construction
  arc A65 (-183.5719, 23.3296) -> (-185.6932, 25.4509) centre (-185.6932, 23.3296) ccw construction
  spline S273 degree 3 poles (-183.5719, 23.3296) (-183.5719, 22.4716) (-184.0887, 21.6981) (-184.8814, 21.3698) knots 0 0 0 0 1 1 1 1 construction
  spline S274 degree 3 poles (-184.8814, 21.3698) (-185.6741, 21.0414) (-186.5865, 21.2229) (-187.1932, 21.8296) knots 0 0 0 0 1 1 1 1 construction
  arc A66 (-174.1739, 4.2796) -> (-176.2952, 6.4009) centre (-176.2952, 4.2796) ccw construction
  spline S275 degree 3 poles (-174.1739, 4.2796) (-174.1739, 3.4216) (-174.6907, 2.6481) (-175.4834, 2.3198) knots 0 0 0 0 1 1 1 1 construction
  spline S276 degree 3 poles (-175.4834, 2.3198) (-176.2761, 1.9914) (-177.1885, 2.1729) (-177.7952, 2.7796) knots 0 0 0 0 1 1 1 1 construction
  spline S277 degree 3 poles (-177.7952, 2.7796) (-178.4019, 3.3863) (-178.5834, 4.2987) (-178.255, 5.0914) knots 0 0 0 0 1 1 1 1 construction
  spline S278 degree 3 poles (-178.255, 5.0914) (-177.9267, 5.8841) (-177.1532, 6.4009) (-176.2952, 6.4009) knots 0 0 0 0 1 1 1 1 construction
  spline S279 degree 3 poles (-158.4654, 50.0266) (-159.2581, 49.6982) (-160.1705, 49.8797) (-160.7772, 50.4864) knots 0 0 0 0 1 1 1 1 construction
  spline S280 degree 3 poles (-160.7772, 50.4864) (-161.3839, 51.0931) (-161.5654, 52.0055) (-161.237, 52.7982) knots 0 0 0 0 1 1 1 1 construction
  spline S281 degree 3 poles (-161.237, 52.7982) (-160.9087, 53.5909) (-160.1352, 54.1077) (-159.2772, 54.1077) knots 0 0 0 0 1 1 1 1 construction
  arc A67 (-157.1559, 51.9864) -> (-159.2772, 54.1077) centre (-159.2772, 51.9864) ccw construction
  spline S282 degree 3 poles (-157.1559, 51.9864) (-157.1559, 51.1284) (-157.6727, 50.3549) (-158.4654, 50.0266) knots 0 0 0 0 1 1 1 1 construction
  spline S283 degree 3 poles (-155.1239, 4.2796) (-155.1239, 3.4216) (-155.6407, 2.6481) (-156.4334, 2.3198) knots 0 0 0 0 1 1 1 1 construction
  spline S284 degree 3 poles (-156.4334, 2.3198) (-157.2261, 1.9914) (-158.1385, 2.1729) (-158.7452, 2.7796) knots 0 0 0 0 1 1 1 1 construction